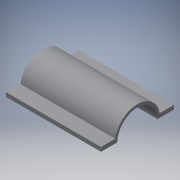
# Autodesk Inventor part: attachment
Saved by Autodesk Inventor 2016 SP1 (Build 200210100, 210)
## iProperties
Created: 2016-04-06
Part Number: attachment
Material: Generic
Document SubType Name: Modeling
Designer: jmehta38
Density: 1 g/cm^3
Appearance: Default
Author: jmehta38
Autodesk Inventor part; units mm, degrees
ref_plane "YZ Plane" through (0, 0, 0) normal (1, 0, 0) x (0, 1, 0)
ref_plane "XZ Plane" through (0, 0, 0) normal (0, 1, 0) x (-1, 0, 0)
ref_plane "XY Plane" through (0, 0, 0) normal (0, 0, 1) x (1, 0, 0)
sketch "Sketch1" plane through (0, 0, 0) normal (1, 0, 0) x (0, 1, 0)
  arc A0 (0, -25) -> (0, 0) centre (0, -12.5) ccw
  arc A1 (2.54, -26.27) -> (2.54, 1.27) centre (0.3727, -12.5) ccw
  line L0 (0, 0) -> (-0.4318, 0)
  line L1 (-0.4318, 0) -> (-0.4318, 10.16)
  line L2 (-0.4318, 10.16) -> (2.54, 10.16)
  line L3 (2.54, 10.16) -> (2.54, 1.27)
  line L4 (2.54, 1.27) -> (2.54, 1.27)
  line L5 (0, -25) -> (-0.4318, -25)
  line L6 (-0.4318, -25) -> (-0.4318, -35.16)
  line L7 (-0.4318, -35.16) -> (2.54, -35.16)
  line L8 (2.54, -35.16) -> (2.54, -26.27)
  line L9 (2.54, -26.27) -> (2.54, -26.27)
  dimension "d0" = 25
  dimension "d9" = 13.77
  dimension "d11" = 12.5
  dimension "d41" = 10.16
  dimension "d45" = 10.16
  dimension "d47" = 1.27
  dimension "d48" = 1.27
  dimension "d50" = 13.9395
  dimension "d52" = 0.3727
  dimension "d54" = 0
  dimension "d55" = 0
  constraints: 20 end point, 6 perpendicular, 4 point on circle, 2 centre point, 2 horizontal, 2 vertical
  measures "d0" distance of L0.start L5.start
  measures "d9" vertical distance of A0.centre L4.end
  measures "d11" radius of A0
  measures "d41" distance of L0.end L1.end
  measures "d45" distance of L5.end L6.end
  measures "d47" distance between parallel lines of L0 L4
  measures "d48" distance between parallel lines of L5 L9
  measures "d50" radius of A1
  measures "d52" distance of A0.centre A1.centre
  measures "d54" distance of L3.end L4.end
  measures "d55" distance of L8.end L9.end
extrude "Extrusion1" add sketch "Sketch1" along normal blind 59
body "Solid1"
